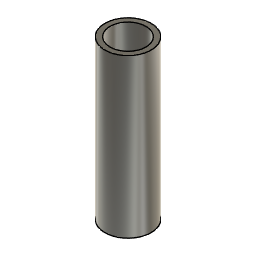
long_rod (Autodesk Fusion 360 design; units mm, degrees)
Autodesk Fusion 360 part; units mm, degrees
sketch "Sketch1" plane through (0, 0, 0) normal (0, 0, 1) x (1, 0, 0)
  circle A0 centre (0, 0) radius 7.75
  dimension "d1" = 15.5
  constraint coincident A0.centre origin
  measures "d1" diameter of A0
extrude "Extrude1" add sketch "Sketch1" along normal blind 27.9
sketch "Sketch2" plane through (0, 0, 27.9) normal (0, 0, 1) x (-1, 0, 0)
  circle A0 centre (0, 0) radius 7.75
  circle A1 centre (0, 0) radius 6
  dimension "d4" = 12
  constraint concentric A0 A1
  measures "d4" diameter of A1
extrude "Extrude2" cut sketch "Sketch2" against normal blind 30 contours A1
extrude "Extrude3" add 1 faces at (7.1155, -0.6831, 27.9) along direction (0, 0, 1) blind 15
extrude "Extrude4" add 1 faces at (7.1155, -0.6831, 42.9) along direction (0, 0, 1) blind 10
